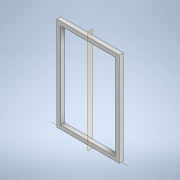
# Autodesk Inventor part: primativeBaseForShortRobot
Saved by Autodesk Inventor 2020.2 (Build 242310000, 310)
## iProperties
Created: 2020-01-09
Part Number: primativeBaseForShortRobot
Material: Generic
Document SubType Name: Modeling
Designer: steele
Density: 1 g/cm^3
Appearance: Default
Author: steele
Autodesk Inventor part; units mm, degrees
ref_plane "XZ Plane" through (0, 0, 0) normal (0, 1, 0) x (-1, 0, 0)
ref_plane "XY Plane" through (0, 0, 0) normal (0, 0, 1) x (1, 0, 0)
sketch "Sketch1" plane through (0, 0, 0) normal (0, 0, 1) x (1, 0, 0)
  line L0 (0, 0) -> (203.2, 0)
  line L1 (203.2, 0) -> (203.2, 609.6)
  line L2 (203.2, 609.6) -> (0, 609.6)
  line L3 (0, 0) -> (0, 609.6) construction
  line L4 (0, 0) -> (-203.2, 0)
  line L5 (-203.2, 0) -> (-203.2, 609.6)
  line L6 (-203.2, 609.6) -> (0, 609.6)
  line L7 (-177.8, 25.4) -> (177.8, 25.4)
  line L8 (177.8, 25.4) -> (177.8, 584.2)
  line L9 (177.8, 584.2) -> (-177.8, 584.2)
  line L10 (-177.8, 584.2) -> (-177.8, 25.4)
  dimension "d1" = 609.6
  dimension "d2" = 406.4
  dimension "d3" = 25.4
  dimension "d4" = 25.4
  dimension "d5" = 25.4
  dimension "d6" = 25.4
  constraints: 22 end point, 3 parallel, 2 horizontal, 2 perpendicular, 2 symmetric about line, 1 vertical
  measures "d1" distance of L1.end L0.end
  measures "d2" distance between parallel lines of L1 L5
  measures "d3" distance between parallel lines of L7 L0
  measures "d4" distance between parallel lines of L1 L8
  measures "d5" distance between parallel lines of L2 L9
  measures "d6" distance between parallel lines of L5 L10
extrude "Extrusion1" add sketch "Sketch1" along normal mid plane 25.4
body "Solid1"
